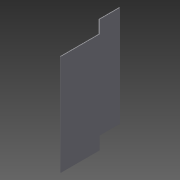
# Autodesk Inventor part: ElectronicsCover1
Saved by Autodesk Inventor 2015 (Build 190159000, 159)
## iProperties
Created: 2014-08-27
Part Number: ElectronicsCover1
Material: Generic
Document SubType Name: Modeling
Designer: t_clevj
Density: 1 g/cm^3
Appearance: Default
Author: t_clevj
Autodesk Inventor part; units mm, degrees
ref_plane "YZ Plane" through (0, 0, 0) normal (1, 0, 0) x (0, 1, 0)
ref_plane "XZ Plane" through (0, 0, 0) normal (0, 1, 0) x (-1, 0, 0)
ref_plane "XY Plane" through (0, 0, 0) normal (0, 0, 1) x (1, 0, 0)
sketch "Sketch1" plane through (0, 0, 0) normal (0, 0, 1) x (1, 0, 0)
  line L0 (0, 0) -> (0, 150)
  line L1 (0, 150) -> (-50, 200)
  line L2 (-50, 200) -> (-50, 280)
  line L3 (-47, 280) -> (-47, 201.2426)
  line L4 (-47, 201.2426) -> (3, 151.2426)
  line L5 (3, 151.2426) -> (3, 0)
  line L6 (-50, 280) -> (-47, 280)
  line L7 (0, 0) -> (3, 0)
  dimension "d0" = 135
  dimension "d1" = 150
  dimension "d2" = 280
  dimension "d3" = 50
  dimension "d4" = 3
  constraints: 16 end point, 3 parallel, 1 horizontal, 1 vertical, 2 other
  measures "d0" angle of L0 L1
  measures "d1" distance of L0.start L0.end
  measures "d2" vertical distance of L2.end L0.start
  measures "d3" distance between parallel lines of L0 L2
  measures "d4" distance between parallel lines of L2 L3
extrude "Extrusion1" add sketch "Sketch1" along normal blind 390
body "Solid1"
